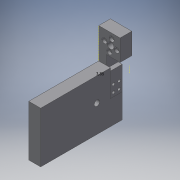
# Autodesk Inventor part: ZnutBracket
Saved by Autodesk Inventor 2019 (Build 230136000, 136)
## iProperties
Created: 2018-10-03
Part Number: ZnutBracket
Material: Generic
Document SubType Name: Modeling
Designer: LillaHunden
Density: 1 g/cm^3
Appearance: Default
Author: LillaHunden
Autodesk Inventor part; units mm, degrees
ref_plane "YZ Plane" through (0, 0, 0) normal (1, 0, 0) x (0, 1, 0)
ref_plane "XZ Plane" through (0, 0, 0) normal (0, 1, 0) x (-1, 0, 0)
ref_plane "XY Plane" through (0, 0, 0) normal (0, 0, 1) x (1, 0, 0)
sketch "Sketch1" plane through (0, 0, 0) normal (0, 0, 1) x (1, 0, 0)
  line L0 (-7.75, 7.8) -> (-7.75, 35.0829)
  line L1 (-7.75, 35.0829) -> (-35.3, 35.0829)
  line L2 (-35.3, 35.0829) -> (-35.3, -38.4359)
  line L3 (-35.3, -38.4359) -> (-20.05, -38.4359)
  line L4 (-20.05, -38.4359) -> (-20.05, -7.832)
  line L5 (-20.05, -7.832) -> (-25.3, -7.832)
  line L6 (-25.3, -7.832) -> (-25.3, 7.8)
  line L7 (-25.3, 7.8) -> (-7.75, 7.8)
  line L8 (6, -5.5) -> (6, -7.5) construction
  line L9 (6, -7.5) -> (25, -7.5) construction
  line L10 (25, -7.5) -> (25, 7.5) construction
  line L11 (25, 7.5) -> (7.55, 7.5) construction
  line L12 (7.55, 7.5) -> (7.55, 2.5) construction
  line L13 (7.55, 2.5) -> (-7.55, 2.5) construction
  line L14 (-7.55, 2.5) -> (-7.55, 7.5) construction
  line L15 (-7.55, 7.5) -> (-25, 7.5) construction
  line L16 (-25, 7.5) -> (-25, -7.5) construction
  line L17 (-25, -7.5) -> (-6, -7.5) construction
  line L18 (-6, -7.5) -> (-6, -5.5) construction
  line L19 (-6, -5.5) -> (6, -5.5) construction
  line L20 (-7.45, 15.5) -> (7.55, 15.5) construction
  line L21 (-7.45, 2.5) -> (-7.45, 15.5) construction
  line L22 (7.55, 2.5) -> (-7.45, 2.5) construction
  line L23 (7.55, 2.5) -> (7.55, 15.5) construction
  line L24 (20, -18.5) -> (-20, -18.5) construction
  line L25 (-20, -18.5) -> (-20, -28.5) construction
  line L26 (20, -28.5) -> (-20, -28.5) construction
  line L27 (20, -18.5) -> (20, -28.5) construction
  line L28 (280, -28.5) -> (-20, -28.5) construction
  line L29 (-20, -28.5) -> (-20, -38.5) construction
  line L30 (280, -38.5) -> (-20, -38.5) construction
  line L31 (280, -28.5) -> (280, -38.5) construction
  point P0 (0, 0)
  dimension "d5" = 0.3
  dimension "d6" = 0.3
  dimension "d7" = 0.3
  dimension "d8" = 10
  dimension "d9" = 0.05
  constraints: 16 end point, 7 perpendicular, 1 vertical
  measures "d5" distance between parallel lines of L16 L6
  measures "d6" distance between parallel lines of L15 L7
  measures "d7" distance between parallel lines of L21 L0
  measures "d8" distance between parallel lines of L6 L2
  measures "d9" distance between parallel lines of L29 L4
extrude "Extrusion1" add sketch "Sketch1" along normal blind 15
sketch "Sketch2" plane through (0, 0, 15) normal (0, 0, 1) x (1, 0, 0)
  circle A0 centre (-20.1, 20.7) radius 5.15 construction
  circle A1 centre (-20.1, 20.7) radius 4.2
  point P0 (0, 0)
  dimension "d18" = 8.4
  constraints: 1 centre point
  measures "d18" diameter of A1
extrude "Extrusion2" cut sketch "Sketch2" against normal through all
sketch "Sketch3" plane through (-35.3, -38.4359, 0) normal (-1, 0, 0) x (0, 0, 1)
  line L0 (-25, 9.9359) -> (-25, -0.0641) construction
  line L1 (40, 19.9359) -> (40, 9.9359) construction
  line L2 (0, 0) -> (15, 0) construction
  line L3 (7.5, 0) -> (7.5, 20.6038) construction
  line L4 (15, 73.5188) -> (15, 0) construction
  point P0 (0, 38.4359)
  point P1 (11.1484, 4.9359)
  point P2 (3.8516, 4.9359)
  point P3 (11.15, 14.1056)
  point P4 (3.85, 14.1056)
  dimension "d10" = 3.85
  constraints: 2 end point, 2 symmetric about line, 1 midpoint, 1 vertical
  measures "d10" distance from line of L4 point (11.15, 14.106)
sketch "Sketch4" plane through (-35.3, -38.4359, 0) normal (-1, 0, 0) x (0, 0, 1)
  point P0 (11.1484, 4.9359)
  point P1 (3.8516, 4.9359)
  point P2 (11.15, 14.1056)
  point P3 (3.85, 14.1056)
hole "Hole1" at (-35.3, -33.5, 11.1484) at (-35.3, -33.5, 3.8516) at (-35.3, -24.3303, 11.15) at (-35.3, -24.3303, 3.85) direction (1, 0, 0) diameter 3.4 depth 15.25 counterbore diameter 6.5 counterbore depth 3.4
sketch "Sketch6" plane through (0, 0, 15) normal (0, 0, 1) x (1, 0, 0)
  point P0 (-27.9739, 22.1148)
  point P1 (-18.6852, 28.5739)
  point P2 (-12.2261, 19.2852)
  point P3 (-21.5148, 12.8261)
hole "Hole3" at (-27.9739, 22.1148, 15) at (-18.6852, 28.5739, 15) at (-12.2261, 19.2852, 15) at (-21.5148, 12.8261, 15) direction (0, 0, -1) diameter 3.4 depth 15 counterbore diameter 6.5 counterbore depth 3.4
sketch "Sketch7" plane through (-35.3, -38.4359, 0) normal (-1, 0, 0) x (0, 0, 1)
  line L0 (15, 73.5188) -> (15, 0) projected
  line L1 (15, 0) -> (45.4011, 0)
  line L2 (45.4011, 0) -> (45.4011, 34.139)
  line L3 (45.4011, 34.139) -> (15, 34.139)
  line L4 (15, 34.139) -> (15, 0)
  line L5 (0, 73.5188) -> (0, 0) projected
  line L6 (0, 0) -> (45.4011, 0)
  line L7 (45.4011, 0) -> (45.4011, -7.6901)
  line L8 (45.4011, -7.6901) -> (0, -7.6901)
  line L9 (0, -7.6901) -> (0, 0)
  point P0 (0, 38.4359)
  constraints: 16 end point, 4 parallel, 2 horizontal, 2 perpendicular, 1 point on line
ref_plane "Work Plane1" through (-20, -38.5, -25) normal (-1, 0, 0) x (0, 0, 1)
extrude "Extrusion3" add sketch "Sketch7" against normal up to surface (15.25 mm away)
sketch "Sketch8" plane through (-35.3, 35.0829, 0) normal (-1, 0, 0) x (0, 0, 1)
  circle A0 centre (32.5096, -69.8259) radius 2.5 construction
  circle A1 centre (32.5096, -69.8259) radius 3.5
  point P0 (0, -35.0829)
  dimension "d28" = 7
  constraints: 1 centre point, 1 coincident
  measures "d28" diameter of A1
extrude "Extrusion4" cut sketch "Sketch8" against normal through all
sketch "Sketch9" plane through (-35.3, 35.0829, 0) normal (-1, 0, 0) x (0, 0, 1)
  circle A0 centre (32.5096, -69.8259) radius 3.5 projected
  circle A1 centre (32.5096, -69.8259) radius 10
  point P0 (0, -35.0829)
  dimension "d31" = 20
  constraints: 1 centre point, 1 coincident
  measures "d31" diameter of A1
extrude "Extrusion5" cut sketch "Sketch9" against normal blind 7.5
sketch "Sketch10" plane through (-35.3, 35.0829, 0) normal (-1, 0, 0) x (0, 0, 1)
  line L0 (45.4011, -39.3798) -> (15, -39.3798) projected
  line L1 (45.4011, -39.3798) -> (104.8234, -39.3798)
  line L2 (104.8234, -39.3798) -> (104.8234, -112.1071)
  line L3 (104.8234, -112.1071) -> (45.4011, -112.1071)
  line L4 (45.4011, -112.1071) -> (45.4011, -39.3798)
  line L5 (0, 0) -> (0, -81.2089) projected
  line L6 (0, -81.2089) -> (45.4011, -81.2089)
  line L7 (45.4011, -81.2089) -> (45.4011, -112.1071)
  line L8 (45.4011, -112.1071) -> (0, -112.1071)
  line L9 (0, -112.1071) -> (0, -81.2089)
  point P0 (0, -35.0829)
  constraints: 16 end point, 4 parallel, 2 horizontal, 2 perpendicular
extrude "Extrusion6" add sketch "Sketch10" against normal up to surface (15.25 mm away)
sketch "Sketch11" plane through (-35.3, 35.0829, 0) normal (-1, 0, 0) x (0, 0, 1)
  circle A0 centre (95.0366, -105.4255) radius 2.5 construction
  circle A1 centre (95.0366, -58.2855) radius 2.75 construction
  circle A2 centre (47.8966, -105.4255) radius 2.5 construction
  circle A3 centre (47.8966, -58.2855) radius 2.75 construction
  circle A4 centre (95.0366, -105.4255) radius 2.75 construction
  circle A5 centre (95.0366, -58.2855) radius 2.5 construction
  point P0 (0, -35.0829)
hole "Hole5" at (-35.3, -23.2026, 95.0366) at (-35.3, -70.3426, 95.0366) at (-35.3, -70.3426, 47.8966) at (-35.3, -23.2026, 47.8966) direction (1, 0, 0) diameter 3.242 depth 11.8 tip angle 118 thread size "M4x0.7" class "6H" standard "ISO Metric profile"
body "Solid1"
